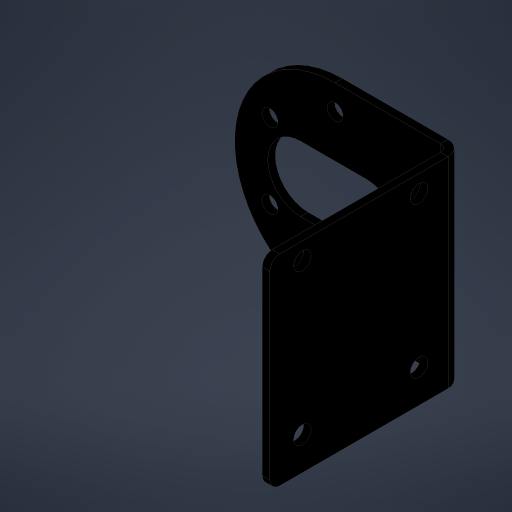
# Autodesk Inventor part: staffa motore
Saved by Autodesk Inventor 2023.1 (Build 271208000, 208)
## iProperties
Created: 2023-11-02
Part Number: staffa motore
Material: Generico
Document SubType Name: Sheet Metal
Designer: never
Density: 1 g/cm^3
Sheet Metal Rule: Default_mm
Appearance: Default
Author: never
Autodesk Inventor part; units mm, degrees
ref_plane "YZ Plane" through (0, 0, 0) normal (1, 0, 0) x (0, 1, 0)
ref_plane "XZ Plane" through (0, 0, 0) normal (0, 1, 0) x (-1, 0, 0)
ref_plane "XY Plane" through (0, 0, 0) normal (0, 0, 1) x (1, 0, 0)
sketch "Schizzo1" plane through (0, 0, 0) normal (0, 0, 1) x (1, 0, 0)
  line L0 (0, -20) -> (-22.5, -20)
  line L1 (-42.5, -20) -> (-42.5, 0)
  line L2 (-22.5, 20) -> (0, 20)
  line L3 (42.5, -20) -> (-42.5, 20) construction
  line L4 (-42.5, -20) -> (42.5, 20) construction
  arc A0 (-22.5, 20) -> (-22.5, -20) centre (-22.5, 0) ccw
  arc A1 (-2.5356, -1.1932) -> (-2.5356, 1.1932) centre (-22.5, 0) ccw
  line L5 (0, 20) -> (0, -20)
  point P0 (0, 0)
  dimension "d1" = 40
  dimension "d2" = 20
  measures "d1" distance of L1.start L3.end
  measures "d2" distance from line of L1 A0.centre
extrude "Piano1" add sketch "Schizzo1" along normal blind 1.5
sketch "Schizzo2" plane through (0, 0, 1.5) normal (0, 0, 1) x (1, 0, 0)
  line L0 (-22.5, 20) -> (0, 20) projected
  point P0 (0, 0)
sketch "Schizzo3" plane through (0, 20, 1.5) normal (1, 0, 0) x (0, 1, 0)
  line L0 (-40, 0) -> (0, 0)
  line L1 (0, 0) -> (0, 37)
  line L2 (0, 37) -> (-40, 37)
  line L3 (-40, 37) -> (-40, 0)
  constraints: 6 end point, 1 horizontal, 1 perpendicular, 1 vertical
edge flange "Flangia1" height 38.5 angle 90 thickness 1.5 bend radius 1.5 thickness toward (1, 0, 0) relief tear relief width 1.5 relief depth 0.75 edges at (0, 0, 1.5) wall of the first edge with corners at (0, -20, 1.5) (0, 20, 1.5) (0, 20, 38.5) (0, -20, 38.5)
bend "Piega (Bend)1"
corner "Angolo1"
sketch "Schizzo4" plane through (1.5, -20, 38.5) normal (1, 0, 0) x (0, 0, -1)
  circle A0 centre (6.5, 36.55) radius 1.75
  line L0 (0, 0) -> (0, 40) projected
  line L1 (0, 40) -> (35.5, 40) projected
  circle A1 centre (29.75, 36.55) radius 1.75
  circle A2 centre (6.5, 6.55) radius 1.75
  circle A3 centre (29.75, 6.55) radius 1.75
  point P0 (38.5, 20)
  dimension "d15" = 3.5
  dimension "d16" = 6.5
  dimension "d17" = 3.45
  dimension "d18" = 3.5
  dimension "d19" = 23.25
  dimension "d20" = 3.5
  dimension "d21" = 30
  dimension "d22" = 3.5
  constraints: 4 centre point
  measures "d15" diameter of A0
  measures "d16" distance from line of L0 A0.centre
  measures "d17" distance from line of L1 A0.centre
  measures "d18" diameter of A1
  measures "d19" distance of A1.centre A0.centre
  measures "d20" diameter of A2
  measures "d21" distance of A2.centre A0.centre
  measures "d22" diameter of A3
hole "Foro1" at (1.5, 16.55, 32) at (1.5, 16.55, 8.75) at (1.5, -13.45, 8.75) at (1.5, -13.45, 32) direction (-1, 0, 0) diameter 3.5 depth 1.5 tip angle 118
sketch "Schizzo5" plane through (0, 0, 0) normal (0, 0, -1) x (-1, 0, 0)
  line L0 (16.15, 0) -> (29.4, 0) construction
  line L1 (16.15, -6.5) -> (29.4, -6.5)
  line L2 (29.4, 6.5) -> (16.15, 6.5)
  arc A0 (16.15, 6.5) -> (16.15, -6.5) centre (16.15, 0) ccw
  arc A1 (29.4, -6.5) -> (29.4, 6.5) centre (29.4, 0) ccw
  arc A2 (22.5, -20) -> (22.5, 20) centre (22.5, 0) ccw projected
  circle A3 centre (22.5, -15) radius 1.6
  circle A4 centre (35.4904, -7.5) radius 1.6
  circle A5 centre (35.4904, 7.5) radius 1.6
  circle A6 centre (22.5, 15) radius 1.6
  circle A7 centre (9.5096, 7.5) radius 1.6
  circle A8 centre (9.5096, -7.5) radius 1.6
  point P0 (0, 0)
  point P1 (22.775, 0)
  point P2 (42.5, 0)
  point P3 (35.9, 0)
  dimension "d30" = 13.25
  dimension "d31" = 13
  dimension "d32" = 6.6
  dimension "d33" = 3.2
  dimension "d34" = 15
  dimension "d39" = 360
  constraints: 8 centre point, 8 end point, 6 point on circle, 4 tangent, 1 horizontal, 1 midpoint, 1 parallel, 13 other
  measures "d30" distance of L0.start L0.end
  measures "d31" diameter of A1
  measures "d32" distance of point (42.5, 0) point (35.9, 0)
  measures "d33" diameter of A3
  measures "d34" distance of A2.centre A3.centre
extrude "Taglia1" cut sketch "Schizzo5" against normal blind 1.5
fillet "Arrotondamento angolo1" radius 2 2 edges at (0.75, 20, 38.5) (0.75, -20, 38.5)
equation "\"d28\" = Spessore"
equation "\"d41\" = Spessore"
equation "\"d3\" = Spessore"
equation "\"d5\" = LarghezzaScaricoPiega"
equation "\"d6\" = ProfonditàScaricoPiega"
equation "\"d7\" = ResiduoMinimo"
equation "\"d8\" = RaggioTransizione"
equation "\"d11\" = RaggioPiega"
equation "\"d12\" = DimensioniScaricoAngolo"
equation "\"d13\" = DimensioneGioco"
equation "\"d14\" = Dimensione_raggio_Jacobi"
equation "\"RaggioPiega\" = Spessore"
equation "\"LarghezzaScaricoPiega\" = Spessore"
equation "\"ProfonditàScaricoPiega\" = 0.5 * Spessore"
equation "\"DimensioniScaricoAngolo\" = 4 * Spessore"
equation "\"ResiduoMinimo\" = 2 * Spessore"
equation "\"RaggioTransizione\" = RaggioPiega"
equation "\"Dimensione_raggio_Jacobi\" = RaggioPiega"
equation "\"DimensioneGioco\" = Spessore"
equation "\"Spessore\" = 1.5"
